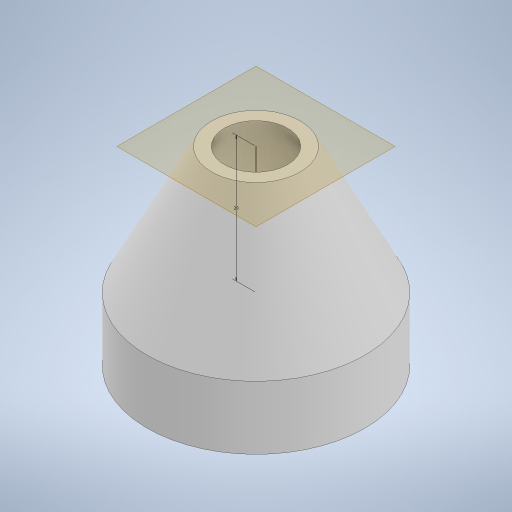
# Autodesk Inventor part: Boquilla
Saved by Autodesk Inventor 2024 (Build 280153000, 153)
## iProperties
Created: 2024-02-26
Part Number: Boquilla
Material: Genérico
Document SubType Name: Modeling
Designer: Juan David
Density: 1 g/cm^3
Appearance: Valor por defecto
Author: Juan David
Autodesk Inventor part; units mm, degrees
ref_plane "YZ Plane" through (0, 0, 0) normal (1, 0, 0) x (0, 1, 0)
ref_plane "XZ Plane" through (0, 0, 0) normal (0, 1, 0) x (-1, 0, 0)
ref_plane "XY Plane" through (0, 0, 0) normal (0, 0, 1) x (1, 0, 0)
sketch "Boceto2" plane through (0, 0, 0) normal (0, 0, 1) x (1, 0, 0)
  line L0 (0, 0) -> (0, 20)
  dimension "d2" = 20
  constraints: 2 end point, 1 vertical
  measures "d2" distance of L0.start L0.end
ref_plane "Plano de trabajo1" through (0, 20, 0) normal (0, 1, 0) x (-1, 0, 0)
sketch "Boceto4" plane through (0, 20, 0) normal (0, 1, 0) x (-1, 0, 0)
  circle A0 centre (0, 0) radius 5
  circle A1 centre (0, 0) radius 7
  dimension "d13" = 10
  dimension "d14" = 14
  constraints: 2 centre point, 2 coincident
  measures "d13" diameter of A0
  measures "d14" diameter of A1
extrude "Extrusión1" add sketch "Boceto4" against normal blind 20 draft 27
sketch "Boceto7" plane through (0, 20, 0) normal (0, 1, 0) x (1, 0, 0)
  circle A0 centre (0, 0) radius 7 projected
  circle A1 centre (0, 0) radius 5
  constraints: 1 centre point, 1 coincident
extrude "Extrusión2" cut sketch "Boceto7" against normal blind 20 draft 24 contours A1
sketch "Boceto9" plane through (0, 0, 0) normal (0, -1, 0) x (1, 0, 0)
  circle A0 centre (0, 0) radius 13.9046 projected
  circle A1 centre (0, 0) radius 13.9046
  circle A2 centre (0, 0) radius 17.1905
  constraints: 2 centre point, 2 coincident
extrude "Extrusión3" add sketch "Boceto9" along normal blind 10
